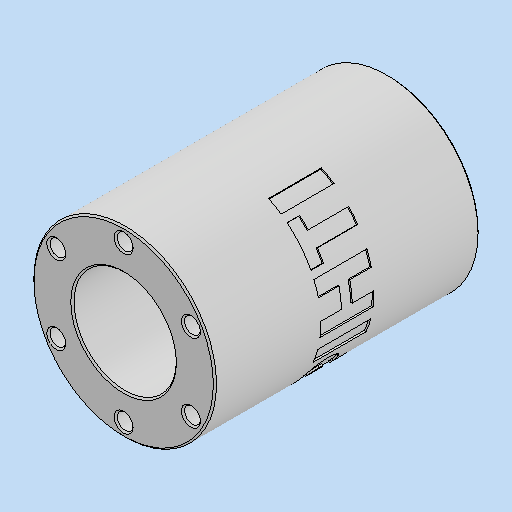
# Autodesk Inventor part: Cathode-Flange-Stand
Saved by Autodesk Inventor 2025 (Build 290162000, 162)
## iProperties
Created: 2024-11-14
Part Number: Cathode-Flange-Stand
Material: Generic
Document SubType Name: Modeling
Designer: kuzmin
Density: 1 g/cm^3
Appearance: Default
Author: kuzmin
Autodesk Inventor part; units mm, degrees
ref_plane "XZ Plane" through (0, 0, 0) normal (0, 1, 0) x (-1, 0, 0)
ref_plane "XY Plane" through (0, 0, 0) normal (0, 0, 1) x (1, 0, 0)
sketch "Sketch1" plane through (0, 0, 0) normal (0, 0, 1) x (1, 0, 0)
  circle A0 centre (0, 0) radius 19.35
  circle A1 centre (0, 0) radius 34.5
  dimension "d0" = 69
  dimension "d1" = 38.7
  constraints: 2 centre point, 2 coincident
  measures "d0" diameter of A1
  measures "d1" diameter of A0
extrude "Extrusion1" add sketch "Sketch1" along normal blind 100
sketch "Sketch2" plane through (0, 0, 100) normal (0, 0, 1) x (1, 0, 0)
  circle A0 centre (0, 0) radius 29.35 construction
  point P0 (0, -29.35)
  dimension "d4" = 58.7
  constraints: 2 vertical alignment, 1 coincident, 2 other
hole "Hole1" at (0, -29.35, 100) direction (0, 0, -1) diameter 6 depth 20 tip angle 118
chamfer "Chamfer2" distance 0.6 angle 45 1 edges at (0, -26.35, 100)
pattern_circular "Circular Pattern1" count 6 over 360 about axis through (0, 0, 0) along (0, 0, 1) of "Hole1", "Chamfer2"
ref_plane "Work Plane1" through (34.5, 0, 0) normal (1, 0, 0) x (0, 1, 0)
sketch "Sketch3" plane through (34.5, 0, 0) normal (1, 0, 0) x (0, 1, 0)
  line L0 (-34.5267, 59.9077) -> (34.4733, 60) construction
  line L1 (34.4733, 60) -> (34.5, 40) construction
  line L2 (34.5, 40) -> (-34.5, 39.9077) construction
  line L3 (-34.5, 39.9077) -> (-34.5267, 59.9077) construction
  line L4 (34.5, 100) -> (-34.5, 100) construction
  line L5 (34.5, 0) -> (-34.5, 0) construction
  line L6 (0, 0) -> (0, 100) construction
  line L7 (-27.2602, 39.9174) -> (-32.3824, 39.9106)
  line L8 (-32.3824, 39.9106) -> (-32.4091, 59.9105)
  line L9 (-32.4091, 59.9105) -> (-26.7077, 59.9182)
  spline S0 degree 2 poles (-26.7077, 59.9182) (-23.3774, 59.9226) (-21.9833, 59.5987) knots 0 0 0 1 1 1
  spline S1 degree 2 poles (-21.9833, 59.5987) (-20.6254, 59.2385) (-19.7013, 58.4796) knots 0 0 0 1 1 1
  spline S2 degree 2 poles (-19.7013, 58.4796) (-18.6141, 57.5761) (-18.015, 56.2194) knots 0 0 0 1 1 1
  spline S3 degree 2 poles (-18.015, 56.2194) (-17.434, 54.8446) (-17.4317, 53.1613) knots 0 0 0 1 1 1
  spline S4 degree 2 poles (-17.4317, 53.1613) (-17.4293, 51.3514) (-18.0067, 50.0112) knots 0 0 0 1 1 1
  spline S5 degree 2 poles (-18.0067, 50.0112) (-18.5298, 48.6712) (-19.687, 47.7828) knots 0 0 0 1 1 1
  spline S6 degree 2 poles (-19.687, 47.7828) (-20.5187, 47.1301) (-21.6948, 46.8389) knots 0 0 0 1 1 1
  spline S7 degree 2 poles (-21.6948, 46.8389) (-22.7442, 46.5479) (-25.3505, 46.5444) knots 0 0 0 1 1 1
  line L10 (-25.3505, 46.5444) -> (-26.2917, 46.5431)
  line L11 (-26.2917, 46.5431) -> (-27.269, 46.5418)
  line L12 (-27.269, 46.5418) -> (-27.2602, 39.9174)
  line L13 (-27.2749, 50.9219) -> (-26.2432, 50.9233)
  spline S8 degree 2 poles (-26.2432, 50.9233) (-24.3066, 50.9259) (-23.4929, 51.4881) knots 0 0 0 1 1 1
  spline S9 degree 2 poles (-23.4929, 51.4881) (-22.7153, 52.014) (-22.717, 53.3172) knots 0 0 0 1 1 1
  spline S10 degree 2 poles (-22.717, 53.3172) (-22.7187, 54.5479) (-24.2405, 55.6319) (-26.1952, 55.6293) knots 0 0 0 1 2 2 2
  line L14 (-26.1952, 55.6293) -> (-27.2812, 55.6278)
  line L15 (-27.2812, 55.6278) -> (-27.2749, 50.9219)
  line L16 (-14.5, 39.9345) -> (-14.5268, 59.9345)
  line L17 (-14.5268, 59.9345) -> (-9.0245, 59.9418)
  line L18 (-9.0245, 59.9418) -> (-8.9978, 39.9418)
  line L19 (-8.9978, 39.9418) -> (-14.5, 39.9345)
  line L20 (-4.5815, 39.9477) -> (-4.6082, 59.9477)
  line L21 (-4.6082, 59.9477) -> (0.8397, 59.955)
  line L22 (0.8397, 59.955) -> (0.8501, 52.1903)
  line L23 (0.8501, 52.1903) -> (8.1261, 52.2)
  line L24 (8.1261, 52.2) -> (8.1157, 59.9647)
  line L25 (8.1157, 59.9647) -> (13.5637, 59.972)
  line L26 (13.5637, 59.972) -> (13.5905, 39.972)
  line L27 (13.5905, 39.972) -> (8.1425, 39.9648)
  line L28 (8.1425, 39.9648) -> (8.1316, 48.1095)
  line L29 (8.1316, 48.1095) -> (0.8556, 48.0998)
  line L30 (0.8556, 48.0998) -> (0.8665, 39.955)
  line L31 (0.8665, 39.955) -> (-4.5815, 39.9477)
  line L32 (20.7398, 39.9816) -> (20.7193, 55.2576)
  line L33 (20.7193, 55.2576) -> (16.2307, 55.2516)
  line L34 (16.2307, 55.2516) -> (16.2243, 59.9756)
  line L35 (16.2243, 59.9756) -> (30.6497, 59.9949)
  line L36 (30.6497, 59.9949) -> (30.656, 55.2709)
  line L37 (30.656, 55.2709) -> (26.1673, 55.2649)
  line L38 (26.1673, 55.2649) -> (26.1877, 39.9889)
  line L39 (26.1877, 39.9889) -> (20.7398, 39.9816)
  line L40 (33.4637, 39.9986) -> (33.437, 59.9986)
  line L41 (33.437, 59.9986) -> (38.9393, 60.006)
  line L42 (38.9393, 60.006) -> (38.966, 40.006)
  line L43 (38.966, 40.006) -> (33.4637, 39.9986)
  point P0 (34.4866, 50)
  point P1 (0, 50)
  point P2 (0, 39.9539)
  dimension "d11" = 20
  constraints: 4 midpoint, 1 horizontal alignment, 1 vertical alignment, 2 other
  measures "d11" distance of L0.end L1.end
emboss "Emboss1" sketch "Sketch3" operation cut depth 0.6 direction (-1, 0, 0) wrap yes faces at (34.0856, -5.3309, 66.6667)
chamfer "Chamfer1" distance 0.6 angle 45 4 edges at (-34.5, 0, 100) (-34.5, 0, 0) (-19.35, 0, 0) (-19.35, 0, 100)
body "Solid1"
